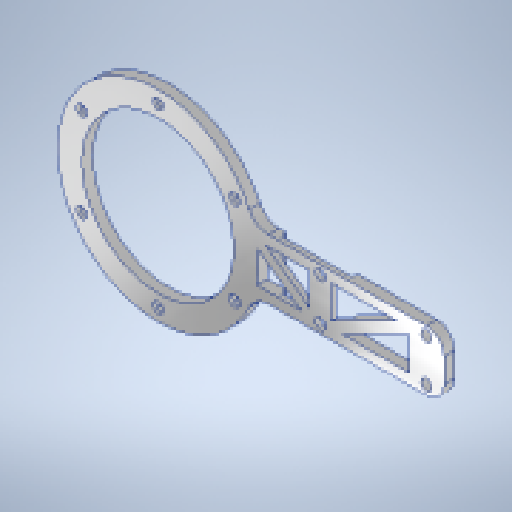
# Autodesk Inventor part: link2plate3
Saved by Autodesk Inventor 2024 (Build 280153000, 153)
## iProperties
Created: 2025-02-10
Part Number: link2plate3
Material: アルミニウム 6061
Document SubType Name: Modeling
Designer: tanoue_kota
Density: 2.7 g/cm^3
Appearance: アルミニウム - フラット
Mass: 11.9351 g
Surface Area: 53.5506 cm^2
Volume: 4.42042 cm^3
Author: tanoue_kota
Autodesk Inventor part; units mm, degrees
ref_plane "YZ Plane" through (0, 0, 0) normal (1, 0, 0) x (0, 1, 0)
ref_plane "XZ Plane" through (0, 0, 0) normal (0, 1, 0) x (-1, 0, 0)
ref_plane "XY Plane" through (0, 0, 0) normal (0, 0, 1) x (1, 0, 0)
sketch "スケッチ1" plane through (0, 0, 0) normal (0, 0, 1) x (1, 0, 0)
  line L0 (0, 0) -> (-109.5, 0)
  line L1 (-109.5, 0) -> (-109.5, 17)
  line L2 (-109.5, 17) -> (0, 17)
  line L3 (0, 17) -> (0, 0)
  line L4 (0, 8.5) -> (-109.5, 8.5)
  circle A0 centre (-81, 8.5) radius 28.5
  point P0 (-53.7971, 17)
  point P1 (-53.7971, 0)
  dimension "d0" = 17
  dimension "d48" = 57
  dimension "d51" = 81
  constraints: 10 end point, 2 midpoint, 2 parallel, 1 centre point, 1 horizontal, 1 perpendicular, 1 point on line, 1 tangent
  measures "d0" distance of L2.end L0.start
  measures "d48" diameter of A0
  measures "d51" distance from line of L3 A0.centre
extrude "押し出し1" add sketch "スケッチ1" along normal blind 3 contours L0 A0 L4 L3 | A0 L0 | L0 A0 L4 | L4 A0 L2 L3 | L4 A0 L2 | L2 A0
sketch "スケッチ2" plane through (0, 0, 3) normal (0, 0, 1) x (1, 0, 0)
  line L0 (0, 17) -> (-53.7971, 17) projected
  line L1 (-5, 17) -> (-5, 0)
  line L2 (-53.7971, 0) -> (0, 0) projected
  line L3 (-35, 17) -> (-35, 0)
  line L4 (0, 0) -> (0, 17) projected
  line L5 (0, 8.5) -> (-5, 8.5)
  line L6 (-35, 17) -> (-53.7971, 17)
  point P0 (-5, 14.5)
  point P1 (-35, 14.5)
  point P2 (-5, 2.5)
  point P3 (-35, 2.5)
  dimension "d4" = 5
  dimension "d5" = 30
  dimension "d49" = 6
  dimension "d50" = 6
  constraints: 8 end point, 4 point on line, 2 midpoint, 2 symmetric about line, 2 vertical, 1 horizontal
  measures "d4" distance between parallel lines of L4 L1
  measures "d5" distance between parallel lines of L1 L3
  measures "d49" distance from line of L5 point (-5, 14.5)
  measures "d50" distance from line of L5 point (-35, 14.5)
hole "穴1" at (-5, 14.5, 3) at (-35, 14.5, 3) at (-5, 2.5, 3) at (-35, 2.5, 3) direction (0, 0, -1) diameter 3.1 depth 20 tip angle 118
sketch "スケッチ7" plane through (0, 0, 0) normal (0, 0, -1) x (-1, 0, 0)
  arc A0 (53.7971, 0) -> (53.7971, 17) centre (81, 8.5) ccw projected
  circle A1 centre (81, 8.5) radius 25
  line L0 (81, 8.5) -> (81, 33.5)
  line L1 (81, 8.5) -> (81, 33.5)
  point P0 (0, 0)
  point P1 (81, 33.5)
  point P2 (59.3494, 21)
  point P3 (59.3494, -4)
  point P4 (81, -16.5)
  point P5 (102.6506, -4)
  point P6 (102.6506, 21)
  dimension "d52" = 50
  dimension "d55" = 360
  dimension "d75" = 0
  constraints: 4 end point, 3 point on circle, 1 centre point, 1 coincident, 1 point on line, 1 vertical, 7 other
  measures "d52" diameter of A1
  measures "d75" distance between parallel lines of L0 L1
hole "穴3" at (-81, 33.5, 0) at (-59.3494, 21, 0) at (-59.3494, -4, 0) at (-81, -16.5, 0) at (-102.6506, -4, 0) at (-102.6506, 21, 0) direction (0, 0, 1) diameter 3.1 end through all
sketch "スケッチ8" plane through (0, 0, 0) normal (0, 0, -1) x (-1, 0, 0)
  arc A0 (53.7971, 0) -> (53.7971, 17) centre (81, 8.5) ccw projected
  circle A1 centre (81, 8.5) radius 21.5
  point P0 (0, 0)
  dimension "d64" = 43
  constraints: 1 centre point, 1 coincident
  measures "d64" diameter of A1
extrude "押し出し5" cut sketch "スケッチ8" against normal blind 3
sketch "スケッチ9" plane through (0, 0, 0) normal (0, 0, -1) x (-1, 0, 0)
  circle A0 centre (59.3494, -4) radius 1.55 projected
  circle A1 centre (59.3494, -4) radius 3
  circle A2 centre (59.3494, 21) radius 1.55 projected
  circle A3 centre (59.3494, 21) radius 3
  circle A4 centre (81, 33.5) radius 1.55 projected
  circle A5 centre (81, 33.5) radius 3
  circle A6 centre (102.6506, 21) radius 1.55 projected
  circle A7 centre (102.6506, 21) radius 3
  circle A8 centre (102.6506, -4) radius 1.55 projected
  circle A9 centre (102.6506, -4) radius 3
  circle A10 centre (81, -16.5) radius 1.55 projected
  circle A11 centre (81, -16.5) radius 3
  point P0 (0, 0)
  dimension "d67" = 6
  dimension "d68" = 6
  dimension "d69" = 6
  dimension "d70" = 6
  dimension "d71" = 6
  dimension "d72" = 6
  constraints: 6 centre point, 6 coincident
  measures "d67" diameter of A1
  measures "d68" diameter of A3
  measures "d69" diameter of A5
  measures "d70" diameter of A7
  measures "d71" diameter of A9
  measures "d72" diameter of A11
extrude "押し出し6" cut sketch "スケッチ9" against normal blind 2 contours A1 | A2 | A3 | A4 | A5 | A6 | A7 | A8 | A9 | A10 | A11
sketch "スケッチ10" plane through (0, 0, 0) normal (0, 0, -1) x (-1, 0, 0)
  line L0 (0, 17) -> (53.7971, 17) projected
  line L1 (10, 17) -> (10, 0)
  line L2 (0, 0) -> (0, 17) projected
  line L3 (53.7971, 0) -> (0, 0) projected
  line L4 (32, 17) -> (38, 17)
  line L5 (38, 17) -> (38, 0)
  line L6 (38, 0) -> (32, 0)
  line L7 (32, 0) -> (32, 17)
  line L8 (10, 3) -> (53.0357, 3)
  line L9 (10, 14) -> (38, 14)
  arc A0 (53.7971, 0) -> (53.7971, 17) centre (81, 8.5) ccw projected
  circle A1 centre (81, 8.5) radius 28.5
  line L10 (38, 14) -> (53.0357, 14)
  line L11 (53.0357, 14) -> (38, 3)
  line L12 (50.4953, 14) -> (38, 4.8586)
  line L13 (40.5404, 3) -> (52.7033, 11.8982)
  line L14 (10, 14) -> (32, 3)
  line L15 (13.3541, 14) -> (32, 4.6771)
  line L16 (10, 12.3229) -> (28.6459, 3)
  point P0 (35, 6.5)
  point P1 (32, 14)
  dimension "d76" = 10
  dimension "d77" = 3
  dimension "d78" = 3
  dimension "d79" = 3
  dimension "d80" = 3
  dimension "d81" = 1.5
  dimension "d82" = 1.5
  dimension "d83" = 1.5
  dimension "d84" = 1.5
  constraints: 28 end point, 17 point on line, 5 parallel, 4 point on circle, 3 perpendicular, 2 horizontal, 1 centre point, 1 coincident, 1 vertical
  measures "d76" distance between parallel lines of L2 L1
  measures "d77" distance from line of point (35, 6.5) L7
  measures "d78" distance from line of L5 point (35, 6.5)
  measures "d79" distance between parallel lines of L0 L9
  measures "d80" distance between parallel lines of L3 L8
  measures "d81" distance between parallel lines of L11 L12
  measures "d82" distance between parallel lines of L11 L13
  measures "d83" distance between parallel lines of L14 L15
  measures "d84" distance between parallel lines of L14 L16
extrude "押し出し7" cut sketch "スケッチ10" against normal blind 3 contours L7 L15 L9 | L16 L8 L1 | L10 L12 L5 | L13 A1 L8
fillet "フィレット1" radius 6 2 edges at (-53.7971, 0, 1.5) (-53.7971, 17, 1.5)
fillet "フィレット2" radius 5 2 edges at (0, 17, 1.5) (0, 0, 1.5)
sketch "スケッチ11" plane through (0, 0, 0) normal (0, 0, -1) x (-1, 0, 0)
  line L0 (5, 17) -> (49.695, 17) projected
  line L1 (27.5, 17) -> (47.5, 17)
  line L2 (47.5, 17) -> (47.5, 0)
  line L3 (47.5, 0) -> (27.5, 0)
  line L4 (27.5, 0) -> (27.5, 17)
  line L5 (0, 5) -> (0, 12) projected
  line L6 (47.5, 17) -> (47.5, 17.4159)
  arc A0 (49.695, 17) -> (55.1394, 20.4783) centre (49.695, 23) ccw projected
  line L7 (47.5, 0) -> (47.5, -0.4159)
  arc A1 (55.1394, -3.4783) -> (49.695, 0) centre (49.695, -6) ccw projected
  point P0 (0, 0)
  point P1 (47.5, 17)
  point P2 (46.695, 17)
  dimension "d89" = 27.5
  dimension "d90" = 20
  constraints: 12 end point, 2 parallel, 2 point on circle, 2 point on line, 1 horizontal, 1 perpendicular, 1 vertical
  measures "d89" distance between parallel lines of L5 L4
  measures "d90" distance between parallel lines of L4 L2
extrude "押し出し8" cut sketch "スケッチ11" against normal blind 1.5
